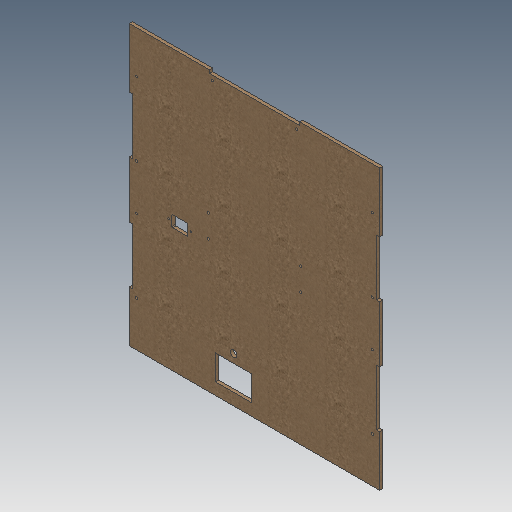
# Autodesk Inventor part: Culata Carcaza
Saved by Autodesk Inventor 2020 (Build 240168000, 168)
## iProperties
Created: 2020-06-26
Part Number: Culata Carcaza
Material: MDF Tablero de fibras de densidad media
Document SubType Name: Modeling
Designer: Pipi
Density: 0.8 g/cm^3
Appearance: Cartón - Ondulado
Author: Pipi
Autodesk Inventor part; units mm, degrees
ref_plane "YZ Plane" through (0, 0, 0) normal (1, 0, 0) x (0, 1, 0)
ref_plane "XZ Plane" through (0, 0, 0) normal (0, 1, 0) x (-1, 0, 0)
ref_plane "XY Plane" through (0, 0, 0) normal (0, 0, 1) x (1, 0, 0)
sketch "Boceto1" plane through (0, 0, 0) normal (0, 1, 0) x (-1, 0, 0)
  line L0 (20.1179, -131.2303) -> (-79.8821, -131.2303)
  line L1 (-79.8821, -131.2303) -> (-79.8821, -125.7303)
  line L2 (-79.8821, -125.7303) -> (-179.8821, -125.7303)
  line L3 (-179.8821, -125.7303) -> (-179.8821, -131.2303)
  line L4 (-179.8821, -131.2303) -> (-279.8821, -131.2303)
  line L5 (-279.8821, -131.2303) -> (-279.8821, -125.7303)
  line L6 (-279.8821, -125.7303) -> (-379.8821, -125.7303)
  line L7 (20.1179, -131.2303) -> (-79.8821, -131.2303)
  line L8 (-179.8821, -131.2303) -> (-279.8821, -131.2303)
  line L9 (25.6179, 11.2697) -> (20.1179, 11.2697)
  line L10 (20.1179, 313.7697) -> (25.6179, 313.7697)
  line L11 (25.6179, 313.7697) -> (25.6179, 171.2697)
  line L12 (25.6179, 171.2697) -> (20.1179, 171.2697)
  line L13 (20.1179, 171.2697) -> (20.1179, 11.2697)
  line L14 (25.6179, 11.2697) -> (25.6179, -131.2303)
  line L15 (25.6179, -131.2303) -> (20.1179, -131.2303)
  line L16 (-379.8821, -125.7303) -> (-379.8821, -131.2303)
  line L17 (-379.8821, -131.2303) -> (-469.8821, -131.2303)
  line L18 (-469.8821, 313.7697) -> (-379.8821, 313.7697)
  line L19 (-379.8821, 313.7697) -> (-379.8821, 308.2697)
  line L20 (-379.8821, 308.2697) -> (-279.8821, 308.2697)
  line L21 (-279.8821, 308.2697) -> (-279.8821, 313.7697)
  line L22 (-279.8821, 313.7697) -> (-179.8821, 313.7697)
  line L23 (-179.8821, 313.7697) -> (-179.8821, 308.2697)
  line L24 (-179.8821, 308.2697) -> (-79.8821, 308.2697)
  line L25 (-79.8821, 308.2697) -> (-79.8821, 313.7697)
  line L26 (-79.8821, 313.7697) -> (25.6179, 313.7697)
  line L27 (-469.8821, -131.2303) -> (-469.8821, 23.2697)
  line L28 (-469.8821, 85.2697) -> (-469.8821, 313.7697)
  line L29 (-469.8821, 23.2697) -> (-469.8821, 85.2697)
  line L30 (-448.8821, 21.7697) -> (-448.8821, 86.7697)
  line L31 (-448.8821, 86.7697) -> (-404.3821, 86.7697)
  line L32 (-404.3821, 86.7697) -> (-404.3821, 21.7697)
  line L33 (-404.3821, 21.7697) -> (-448.8821, 21.7697)
  circle A0 centre (-195.3821, 173.2697) radius 2
  circle A1 centre (-235.3821, 173.2697) radius 2
  circle A2 centre (-235.3821, 9.2697) radius 2
  circle A3 centre (-195.3821, 9.2697) radius 2
  circle A4 centre (-49.3821, 300.5547) radius 2
  circle A5 centre (-179.3821, 300.5547) radius 2
  circle A6 centre (-259.8821, 300.5547) radius 2
  circle A7 centre (-389.8821, 300.5547) radius 2
  circle A8 centre (-49.3821, -118.0153) radius 2
  circle A9 centre (-179.3821, -118.0153) radius 2
  circle A10 centre (-259.8821, -118.0153) radius 2
  circle A11 centre (-389.8821, -118.0153) radius 2
  circle A12 centre (11.6179, 166.2697) radius 2
  circle A13 centre (11.6179, 16.2697) radius 2
  circle A14 centre (-239.8821, -61.2303) radius 1.625
  circle A15 centre (-239.8821, -21.2303) radius 1.625
  line L34 (-231.2821, -54.7803) -> (-248.4821, -54.7803)
  line L35 (-231.2821, -27.6803) -> (-248.4821, -27.6803)
  line L36 (-230.2821, -28.6803) -> (-230.2821, -53.7803)
  circle A16 centre (-389.3821, 54.2697) radius 6
  line L37 (-249.4821, -28.6803) -> (-249.4821, -53.7803)
  arc A17 (-230.2821, -28.6803) -> (-231.2821, -27.6803) centre (-231.2821, -28.6803) ccw
  arc A18 (-231.2821, -54.7803) -> (-230.2821, -53.7803) centre (-231.2821, -53.7803) ccw
  arc A19 (-248.4821, -27.6803) -> (-249.4821, -28.6803) centre (-248.4821, -28.6803) ccw
  arc A20 (-249.4821, -53.7803) -> (-248.4821, -54.7803) centre (-248.4821, -53.7803) ccw
  line L38 (-248.4821, -27.1803) -> (-231.2821, -27.1803)
  arc A21 (-229.7821, -28.6803) -> (-231.2821, -27.1803) centre (-231.2821, -28.6803) ccw
  line L39 (-229.7821, -28.6803) -> (-229.7821, -53.7803)
  arc A22 (-231.2821, -55.2803) -> (-229.7821, -53.7803) centre (-231.2821, -53.7803) ccw
  line L40 (-231.2821, -55.2803) -> (-248.4821, -55.2803)
  arc A23 (-249.9821, -53.7803) -> (-248.4821, -55.2803) centre (-248.4821, -53.7803) ccw
  line L41 (-249.9821, -53.7803) -> (-249.9821, -28.6803)
  arc A24 (-248.4821, -27.1803) -> (-249.9821, -28.6803) centre (-248.4821, -28.6803) ccw
  point P0 (20.1179, 313.7697)
  point P1 (-230.2821, -54.7803)
  point P2 (-249.4821, -54.7803)
  point P3 (-230.2821, -27.6803)
  point P4 (-249.4821, -27.6803)
  dimension "d8" = 445
  dimension "d15" = 5.5
  dimension "d16" = 100
  dimension "d17" = 100
  dimension "d18" = 5.5
  dimension "d26" = 100
  dimension "d52" = 160
  dimension "d53" = 100
  dimension "d54" = 5.5
  dimension "d55" = 90
  dimension "d80" = 4
  dimension "d81" = 274.5
  dimension "d82" = 140.5
  dimension "d85" = 4
  dimension "d87" = 4
  dimension "d94" = 4
  dimension "d95" = 4
  dimension "d96" = 4
  dimension "d97" = 4
  dimension "d98" = 7.715
  dimension "d99" = 75
  dimension "d100" = 130
  dimension "d101" = 7.715
  dimension "d102" = 80
  dimension "d103" = 7.715
  dimension "d104" = 5.5
  dimension "d105" = 130
  dimension "d106" = 7.715
  dimension "d107" = 4
  dimension "d108" = 4
  dimension "d109" = 4
  dimension "d110" = 4
  dimension "d111" = 75
  dimension "d112" = 7.715
  dimension "d113" = 7.715
  dimension "d114" = 130
  dimension "d115" = 7.715
  dimension "d116" = 80
  dimension "d117" = 7.715
  dimension "d118" = 130
  dimension "d119" = 4
  dimension "d120" = 8.5
  dimension "d121" = 4
  dimension "d122" = 8.5
  dimension "d125" = 150
  dimension "d126" = 142.5
  dimension "d127" = 147.5
  dimension "d128" = 40
  dimension "d129" = 4
  dimension "d130" = 40
  dimension "d131" = 274.5
  dimension "d154" = 3.25
  dimension "d155" = 70
  dimension "d156" = 230
  dimension "d157" = 3.25
  dimension "d160" = 19.2
  dimension "d161" = 9.6
  dimension "d167" = 9.6
  dimension "d168" = 19.2
  dimension "d169" = 27.1
  dimension "d171" = 21
  dimension "d177" = 153
  dimension "d178" = 65
  dimension "d179" = 44.5
  constraints: 84 end point, 25 centre point, 16 perpendicular, 16 point on circle, 14 point on line, 8 tangent, 6 horizontal, 4 vertical, 3 parallel, 2 equal radius, 7 other
  measures "d8" distance of L0.start L10.start
  measures "d15" distance of L0.end L1.end
  measures "d16" distance of L1.end L2.end
  measures "d17" distance of L3.end L4.end
  measures "d18" distance of L4.end L5.end
  measures "d26" distance of L0.start L0.end
  measures "d52" distance of L12.end L9.end
  measures "d53" distance of L5.end L6.end
  measures "d54" distance of L6.end L16.end
  measures "d55" distance of L16.end L17.end
  measures "d80" diameter of A0
  measures "d81" distance from line of L28 A0.centre
  measures "d82" distance from line of L22 A0.centre
  measures "d85" diameter of A2
  measures "d87" diameter of A3
  measures "d94" diameter of A4
  measures "d95" diameter of A5
  measures "d96" diameter of A6
  measures "d97" diameter of A7
  measures "d98" distance from line of L24 A4.centre
  measures "d99" distance from line of L11 A4.centre
  measures "d100" distance of A5.centre A4.centre
  measures "d101" distance from line of L24 A5.centre
  measures "d102" distance from line of L28 A7.centre
  measures "d103" distance from line of L20 A7.centre
  measures "d104" distance from line of L18.end L20
  measures "d105" distance of A7.centre A6.centre
  measures "d106" distance from line of L20 A6.centre
  measures "d107" diameter of A8
  measures "d108" diameter of A9
  measures "d109" diameter of A10
  measures "d110" diameter of A11
  measures "d111" distance from line of L14 A8.centre
  measures "d112" distance from line of L2 A8.centre
  measures "d113" distance from line of L2 A9.centre
  measures "d114" distance of A9.centre A8.centre
  measures "d115" distance from line of L6 A11.centre
  measures "d116" distance from line of L27 A11.centre
  measures "d117" distance from line of L6 A10.centre
  measures "d118" distance of A11.centre A10.centre
  measures "d119" diameter of A12
  measures "d120" distance from line of L13 A12.centre
  measures "d121" diameter of A13
  measures "d122" distance from line of L13 A13.centre
  measures "d125" distance of A12.centre A13.centre
  measures "d126" distance of L10.end L11.end
  measures "d127" distance from line of L26 A12.centre
  measures "d128" distance of A1.centre A0.centre
  measures "d129" diameter of A1
  measures "d130" distance of A2.centre A3.centre
  measures "d131" distance from line of L27 A3.centre
  measures "d154" diameter of A14
  measures "d155" distance from line of L4 A14.centre
  measures "d156" distance from line of L27 A14.centre
  measures "d157" diameter of A15
  measures "d160" distance of point (-230.282, -27.68) point (-249.482, -27.68)
  measures "d161" horizontal distance of A15.centre point (-230.282, -27.68)
  measures "d167" horizontal distance of point (-230.282, -54.78) A14.centre
  measures "d168" distance of point (-230.282, -54.78) point (-249.482, -54.78)
  measures "d169" distance of point (-230.282, -27.68) point (-230.282, -54.78)
  measures "d171" distance between parallel lines of L30 L29
  measures "d177" distance between parallel lines of L17 L33
  measures "d178" distance of L31.end L32.end
  measures "d179" distance of L30.end L31.end
extrude "Extrusión1" add sketch "Boceto1" along normal blind 5.5 contours L0 L1 L2 L3 L4 L5 L6 L16 L17 L27 L29 L28 L18 L19 L20 L21 L22 L23 L24 L25 L26 L10 L11 L12 L13 L9 L14 L15
equation "\"d131\" = d81"
